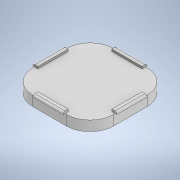
# Autodesk Inventor part: moving_switch(bottom
Saved by Autodesk Inventor 2020 (Build 240168000, 168)
## iProperties
Created: 2020-10-17
Part Number: moving_switch(bottom
Material: 일반
Document SubType Name: Modeling
Designer: KIMJIHUN
Density: 1 g/cm^3
Appearance: 기본값
Author: KIMJIHUN
Autodesk Inventor part; units mm, degrees
ref_plane "YZ Plane" through (0, 0, 0) normal (1, 0, 0) x (0, 1, 0)
ref_plane "XZ Plane" through (0, 0, 0) normal (0, 1, 0) x (-1, 0, 0)
ref_plane "XY Plane" through (0, 0, 0) normal (0, 0, 1) x (1, 0, 0)
sketch "스케치1" plane through (0, 0, 0) normal (0, 1, 0) x (-1, 0, 0)
  line L0 (12, 12) -> (-12, 12)
  line L1 (-12, 12) -> (-12, -12)
  line L2 (-12, -12) -> (12, -12)
  line L3 (12, -12) -> (12, 12)
  point P0 (0, 0)
  dimension "d0" = 24
  dimension "d1" = 24
  dimension "d2" = 12
  dimension "d3" = 12
  constraints: 8 end point, 2 parallel, 1 horizontal, 1 perpendicular
  measures "d0" distance of L2.end L1.end
  measures "d1" distance of L1.end L0.end
  measures "d2" distance from line of L2 point (0, 0)
  measures "d3" distance from line of L1 point (0, 0)
extrude "돌출1" add sketch "스케치1" along normal blind 3
fillet "모깎기1" radius 7 4 edges at (-12, 1.5, 12) (12, 1.5, 12) (12, 1.5, -12) (-12, 1.5, -12)
sketch "스케치2" plane through (0, 3, 0) normal (0, 1, 0) x (1, 0, 0)
  line L0 (12.5, -4.5) -> (-12.5, -4.5)
  line L1 (-12.5, -4.5) -> (-12.5, 4.5)
  line L2 (-12.5, 4.5) -> (12.5, 4.5)
  line L3 (12.5, 4.5) -> (12.5, -4.5)
  line L4 (4.5, -12.5) -> (-4.5, -12.5)
  line L5 (-4.5, -12.5) -> (-4.5, 12.5)
  line L6 (-4.5, 12.5) -> (4.5, 12.5)
  line L7 (4.5, 12.5) -> (4.5, -12.5)
  point P0 (0, 0)
  point P1 (-4.5, -4.5)
  point P2 (-4.5, 4.5)
  point P3 (4.5, -4.5)
  point P4 (4.5, 4.5)
  dimension "d7" = 25
  dimension "d8" = 9
  dimension "d9" = 4.5
  dimension "d10" = 12.5
  dimension "d11" = 9
  dimension "d12" = 25
  dimension "d13" = 12.5
  dimension "d14" = 4.5
  constraints: 16 end point, 4 parallel, 2 horizontal, 2 perpendicular
  measures "d7" distance of L1.end L2.end
  measures "d8" distance of L0.end L1.end
  measures "d9" distance from line of L0 point (0, 0)
  measures "d10" distance from line of L1 point (0, 0)
  measures "d11" distance of L5.end L6.end
  measures "d12" distance of L4.end L5.end
  measures "d13" distance from line of L4 point (0, 0)
  measures "d14" distance from line of L7 point (0, 0)
extrude "돌출2" add sketch "스케치2" along normal blind 0.6 contours L0 L7 L2 L3 | L7 L4 L5 L0 | L0 L1 L2 L5 | L2 L5 L6 L7
fillet "모깎기2" radius 0.6 4 edges at (12.5, 3.6, 0) (0, 3.6, -12.5) (-12.5, 3.6, 0) (0, 3.6, 12.5)
sketch "스케치3" plane through (0, 3.6, 0) normal (0, 1, 0) x (1, 0, 0)
  line L0 (11, -11) -> (-11, -11)
  line L1 (-11, -11) -> (-11, 11)
  line L2 (-11, 11) -> (11, 11)
  line L3 (11, 11) -> (11, -11)
  point P0 (0, 0)
  dimension "d18" = 22
  dimension "d19" = 22
  dimension "d20" = 11
  dimension "d21" = 11
  constraints: 8 end point, 2 parallel, 1 horizontal, 1 perpendicular
  measures "d18" distance of L1.end L2.end
  measures "d19" distance of L0.end L1.end
  measures "d20" distance from line of L1 point (0, 0)
  measures "d21" distance from line of L0 point (0, 0)
extrude "돌출3" cut sketch "스케치3" against normal blind 0.6
sketch "스케치4" plane through (0, 0, 0) normal (0, -1, 0) x (1, 0, 0)
  line L0 (-4.5, 4.5) -> (4.5, 4.5)
  line L1 (4.5, 4.5) -> (4.5, -4.5)
  line L2 (4.5, -4.5) -> (-4.5, -4.5)
  line L3 (-4.5, -4.5) -> (-4.5, 4.5)
  point P0 (0, 0)
  dimension "d24" = 9
  dimension "d25" = 9
  dimension "d26" = 4.5
  dimension "d27" = 4.5
  constraints: 8 end point, 2 parallel, 1 horizontal, 1 perpendicular
  measures "d24" distance of L1.end L2.end
  measures "d25" distance of L0.end L1.end
  measures "d26" distance from line of L0 point (0, 0)
  measures "d27" distance from line of L1 point (0, 0)
extrude "돌출4" add sketch "스케치4" along normal blind 2
sketch "스케치5" plane through (4.5, 0, 4.5) normal (1, 0, 0) x (0, 0, -1)
  line L0 (0.5, -1.5) -> (8.5, -1.5)
  line L1 (8.5, -1.5) -> (8.5, -0.5)
  line L2 (8.5, -0.5) -> (0.5, -0.5)
  line L3 (0.5, -0.5) -> (0.5, -1.5)
  line L4 (0, 0) -> (0, -2) projected
  line L5 (9, -2) -> (0, -2) projected
  point P0 (4.5, 0)
  dimension "d30" = 8
  dimension "d31" = 1
  dimension "d32" = 0.5
  dimension "d33" = 0.5
  constraints: 8 end point, 2 parallel, 1 horizontal, 1 perpendicular
  measures "d30" distance of L2.end L1.end
  measures "d31" distance of L1.end L0.end
  measures "d32" distance between parallel lines of L3 L4
  measures "d33" distance between parallel lines of L5 L0
extrude "돌출5" cut sketch "스케치5" against normal through all
